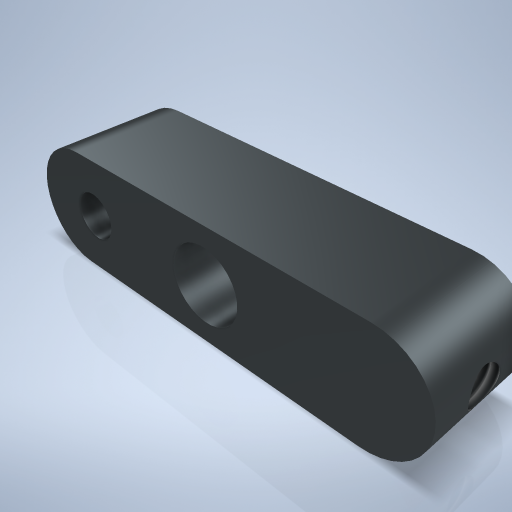
# Autodesk Inventor part: BMS_small
Saved by Autodesk Inventor 2024.2 (Build 282272000, 272)
## iProperties
Created: 2024-05-15
Part Number: BMS_small
Material: Gummi
Document SubType Name: Modeling
Designer: Fabri
Density: 0.93 g/cm^3
Appearance: Eisen - Grau
Author: Fabri
Autodesk Inventor part; units mm, degrees
note: some values were not read from the file. Chosen so that the rebuilt part matches the saved one: direction of "Bohrung1".
ref_plane "XZ Plane" through (0, 0, 0) normal (0, 1, 0) x (-1, 0, 0)
ref_plane "XY Plane" through (0, 0, 0) normal (0, 0, 1) x (1, 0, 0)
sketch "Skizze1" plane through (0, 0, 0) normal (0, 1, 0) x (-1, 0, 0)
  line L0 (14, 0) -> (-14, 0) construction
  line L1 (14, -5) -> (-14, -5)
  line L2 (-14, 5) -> (14, 5)
  arc A0 (14, -5) -> (14, 5) centre (14, 0) ccw
  arc A1 (-14, 5) -> (-14, -5) centre (-14, 0) ccw
  point P0 (0, 0)
  point P1 (0, 0)
  point P2 (-19, 0)
  point P3 (19, 0)
  dimension "d1" = 38
  dimension "d2" = 5
  constraints: 8 end point, 6 point on circle, 4 tangent, 2 centre point, 1 coincident, 1 horizontal, 1 midpoint, 1 parallel
  measures "d1" distance of point (-19, 0) point (19, 0)
  measures "d2" radius of A0
extrude "Extrusion1" add sketch "Skizze1" along normal blind 10
sketch "Skizze2" plane through (0, 10, 0) normal (0, 1, 0) x (1, 0, 0)
  point P0 (0, 0)
  point P1 (0, 0)
  constraints: 1 coincident
hole "Bohrung1" at (0, 10, 0) direction (0, -1, 0) diameter 6.5 depth 10
sketch "Skizze3" plane through (0, 10, 0) normal (0, 1, 0) x (1, 0, 0)
  point P0 (0, 0)
  point P1 (-12.5, 0)
  dimension "d19" = 12.5
  constraints: 1 horizontal alignment
  measures "d19" distance of point (0, 0) point (-12.5, 0)
hole "Bohrung2" at (-12.5, 10, 0) direction (0, -1, 0) diameter 4 end through all
ref_plane "Arbeitsebene1" through (19, 0, 0) normal (1, 0, 0) x (0, 1, 0)
sketch "Skizze4" plane through (19, 0, 0) normal (1, 0, 0) x (0, 1, 0)
  line L0 (0, -5) -> (0, 5) projected
  point P0 (0, 0)
  point P1 (5, 0)
  point P2 (0, 0)
  dimension "d21" = 5
  constraints: 1 horizontal alignment, 1 midpoint
  measures "d21" distance from line of L0 point (5, 0)
hole "Bohrung3" at (19, 5, 0) direction (-1, 0, 0) diameter 3.242 depth 15.75 tip angle 118 thread size "M4x0.7" class "6H" standard "ISO Metric profile"
